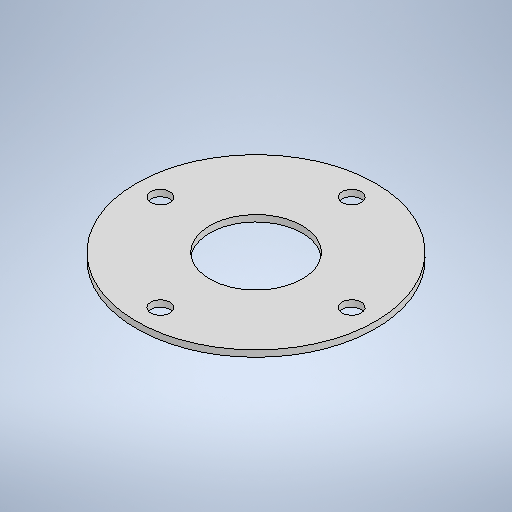
# Autodesk Inventor part: TRM 029 coupling ring
Saved by Autodesk Inventor 2025 (Build 290162010, 162A)
## iProperties
Created: 2024-08-07
Part Number: TRM 029 coupling ring
Material: AISI 304
Document SubType Name: Sheet Metal
Designer: admin
Stock Number: ТРМ 015 левый борт основное
Density: 8.02768 g/cm^3
Flat Pattern Width: 7.5 cm
Flat Pattern Length: 7.5 cm
Flat Pattern Area: 56.25 cm^2
Sheet Metal Rule: AISI304 2mm Die16
Sheet Metal Width: 75,000 mm
Sheet Metal Length: 75,000 mm
Sheet Metal Area: 5625,000 mm^2
Appearance: Default
Author: pokla
Autodesk Inventor part; units mm, degrees
ref_plane "YZ Plane" through (0, 0, 0) normal (1, 0, 0) x (0, 1, 0)
ref_plane "XZ Plane" through (0, 0, 0) normal (0, 1, 0) x (-1, 0, 0)
ref_plane "XY Plane" through (0, 0, 0) normal (0, 0, 1) x (1, 0, 0)
sketch "Sketch1" plane through (0, 0, 0) normal (0, 0, 1) x (1, 0, 0)
  circle A0 centre (0, 0) radius 37.5
  circle A1 centre (0, 0) radius 14.5
  dimension "d15" = 29
  dimension "d16" = 75
  measures "d15" diameter of A1
  measures "d16" diameter of A0
extrude "Plate1" add sketch "Sketch1" along normal blind 2
sketch "Sketch2" plane through (0, 0, 0) normal (0, 0, -1) x (-1, 0, 0)
  line L0 (-27.3167, 25.2399) -> (172.6833, 25.2399) construction
  line L1 (172.6833, 25.2399) -> (172.6833, 5.2399) construction
  line L2 (172.6833, 5.2399) -> (-27.3167, 5.2399) construction
  line L3 (-27.3167, 5.2399) -> (-27.3167, 25.2399) construction
  point P0 (0, 0)
  point P1 (-251, -525)
  dimension "d6" = 200
  dimension "d9" = 20
  constraints: 2 other
  measures "d6" distance of L0.start L0.end
  measures "d9" distance of L0.end L1.end
mark "Mark1"
sketch "Sketch3" plane through (0, 0, 2) normal (0, 0, 1) x (1, 0, 0)
  circle A0 centre (0, 0) radius 14.5 construction
  circle A1 centre (0, 0) radius 37.5 construction
  circle A2 centre (0, 30) radius 3
  line L0 (0, 37.5) -> (0, 14.5) construction
  circle A3 centre (0, 0) radius 30 construction
  dimension "d26" = 60
  dimension "d17" = 6
  dimension "d19" = 7.5
  constraints: 5 vertical alignment, 2 end point, 1 centre point, 1 coincident, 1 vertical, 4 other
  measures "d17" diameter of A2
  measures "d19" distance of L0.start A2.centre
extrude "Cut1" cut sketch "Sketch3" against normal blind 2
pattern_circular "Circular Pattern1" count 4 over 360 about axis through (0, 0, 0) along (0, 0, 1) of "Cut1"
equation "\"d20\" = Thickness"
equation "\"d2\" = Thickness"
equation "\"BendReliefWidth\" = Thickness"
equation "\"BendReliefDepth\" = 0.5 * Thickness"
equation "\"CornerReliefSize\" = 4 * Thickness"
equation "\"MinimumRemnant\" = 2 * Thickness"
equation "\"TransitionRadius\" = BendRadius"
equation "\"JacobiRadiusSize\" = BendRadius"
equation "\"GapSize\" = Thickness"
equation "\"Thickness\" = 2"
equation "\"BendRadius\" = 2.75"
body "Solid1"
